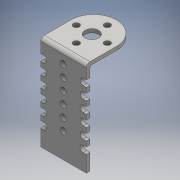
# Autodesk Inventor part: small motor mount
Saved by Autodesk Inventor 2016 (Build 200138000, 138)
## iProperties
Created: 2015-09-29
Part Number: small motor mount
Material: Generic
Document SubType Name: Modeling
Designer: Hulbert Office
Density: 1 g/cm^3
Appearance: Default
Author: Hulbert Office
Autodesk Inventor part; units mm, degrees
ref_plane "YZ Plane" through (0, 0, 0) normal (1, 0, 0) x (0, 1, 0)
ref_plane "XZ Plane" through (0, 0, 0) normal (0, 1, 0) x (-1, 0, 0)
ref_plane "XY Plane" through (0, 0, 0) normal (0, 0, 1) x (1, 0, 0)
sketch "Sketch1" plane through (0, 0, 0) normal (0, 1, 0) x (-1, 0, 0)
  line L0 (0, -52) -> (25, -52)
  line L1 (25, 0) -> (0, 0)
  line L2 (12.5, 0) -> (23.35, 0)
  line L3 (12.5, 0) -> (1.65, 0)
  line L4 (25, -11.25) -> (25, -14.1)
  line L5 (25, -23.95) -> (25, -26.8)
  line L6 (23.35, -7.75) -> (25, -7.75)
  line L7 (23.35, -11.25) -> (25, -11.25)
  arc A0 (23.35, -7.75) -> (23.35, -11.25) centre (23.35, -9.5) ccw
  line L8 (25, 0) -> (25, -7.75)
  arc A1 (23.35, -14.1) -> (23.35, -17.6) centre (23.35, -15.85) ccw
  arc A2 (23.35, -20.45) -> (23.35, -23.95) centre (23.35, -22.2) ccw
  arc A3 (23.35, -26.8) -> (23.35, -30.3) centre (23.35, -28.55) ccw
  arc A4 (23.35, -39.5) -> (23.35, -43) centre (23.35, -41.25) ccw
  line L9 (23.35, -39.5) -> (25, -39.5)
  line L10 (23.35, -43) -> (25, -43)
  line L11 (23.35, -36.65) -> (25, -36.65)
  line L12 (23.35, -33.15) -> (25, -33.15)
  line L13 (23.35, -23.95) -> (25, -23.95)
  line L14 (23.35, -20.45) -> (25, -20.45)
  line L15 (23.35, -17.6) -> (25, -17.6)
  line L16 (23.35, -14.1) -> (25, -14.1)
  line L17 (25, -17.6) -> (25, -20.45)
  line L18 (23.35, -26.8) -> (25, -26.8)
  line L19 (23.35, -30.3) -> (25, -30.3)
  line L20 (25, -43) -> (25, -52)
  line L21 (25, -36.65) -> (25, -39.5)
  arc A5 (23.35, -33.15) -> (23.35, -36.65) centre (23.35, -34.9) ccw
  line L22 (25, -30.3) -> (25, -33.15)
  line L23 (0, -11.25) -> (0, -14.1)
  line L24 (0, -23.95) -> (0, -26.8)
  line L25 (1.65, -7.75) -> (0, -7.75)
  line L26 (1.65, -11.25) -> (0, -11.25)
  arc A6 (1.65, -11.25) -> (1.65, -7.75) centre (1.65, -9.5) ccw
  line L27 (0, 0) -> (0, -7.75)
  arc A7 (1.65, -17.6) -> (1.65, -14.1) centre (1.65, -15.85) ccw
  arc A8 (1.65, -23.95) -> (1.65, -20.45) centre (1.65, -22.2) ccw
  arc A9 (1.65, -30.3) -> (1.65, -26.8) centre (1.65, -28.55) ccw
  arc A10 (1.65, -43) -> (1.65, -39.5) centre (1.65, -41.25) ccw
  line L28 (1.65, -39.5) -> (0, -39.5)
  line L29 (1.65, -43) -> (0, -43)
  line L30 (1.65, -36.65) -> (0, -36.65)
  line L31 (1.65, -33.15) -> (0, -33.15)
  line L32 (1.65, -23.95) -> (0, -23.95)
  line L33 (1.65, -20.45) -> (0, -20.45)
  line L34 (1.65, -17.6) -> (0, -17.6)
  line L35 (1.65, -14.1) -> (0, -14.1)
  line L36 (0, -17.6) -> (0, -20.45)
  line L37 (1.65, -26.8) -> (0, -26.8)
  line L38 (1.65, -30.3) -> (0, -30.3)
  line L39 (0, -43) -> (0, -52)
  line L40 (0, -36.65) -> (0, -39.5)
  arc A11 (1.65, -36.65) -> (1.65, -33.15) centre (1.65, -34.9) ccw
  line L41 (0, -30.3) -> (0, -33.15)
  circle A12 centre (12.5, -6.4) radius 1.65
  circle A13 centre (12.5, -12.75) radius 1.65
  circle A14 centre (12.5, -19.1) radius 1.65
  circle A15 centre (12.5, -25.45) radius 1.65
  circle A16 centre (12.5, -31.8) radius 1.65
  circle A17 centre (12.5, -38.15) radius 1.65
  dimension "d0" = 52
  dimension "d1" = 25
  dimension "d3" = 10.85
  dimension "d27" = 3.5
  dimension "d28" = 3.5
  dimension "d29" = 3.5
  dimension "d31" = 3.5
  dimension "d38" = 3.3
  dimension "d39" = 3.3
  dimension "d40" = 3.3
  dimension "d41" = 3.3
  dimension "d42" = 3.3
  dimension "d43" = 3.3
  constraints: 84 end point, 24 point on circle, 18 centre point, 12 tangent, 7 perpendicular, 2 point on line, 2 vertical, 1 midpoint
  measures "d0" distance of L1.end L0.start
  measures "d1" distance of L0.start L0.end
  measures "d3" distance of L2.start L2.end
  measures "d27" diameter of A1
  measures "d28" diameter of A2
  measures "d29" diameter of A3
  measures "d31" diameter of A4
  measures "d38" diameter of A12
  measures "d39" diameter of A13
  measures "d40" diameter of A14
  measures "d41" diameter of A15
  measures "d42" diameter of A16
  measures "d43" diameter of A17
extrude "Extrusion1" add sketch "Sketch1" along normal blind 2
sketch "Sketch2" plane through (0, 2, 0) normal (0, 1, 0) x (1, 0, 0)
  line L0 (-25, 7.75) -> (-25, 0) projected
  line L1 (-25, 0) -> (-25, 2)
  line L2 (-25, 2) -> (0, 2)
  line L3 (0, 0) -> (0, 7.75) projected
  line L4 (0, 2) -> (0, 0)
  line L5 (-25, 0) -> (0, 0) projected
  line L6 (0, 0) -> (-25, 0)
  dimension "d46" = 2
  constraints: 8 end point, 2 perpendicular, 1 collinear, 1 point on line
  measures "d46" distance of L0.end L1.end
extrude "Extrusion2" add sketch "Sketch2" along normal blind 27
fillet "Fillet1" radius 2 1 edges at (-12.5, 0, 0)
fillet "Fillet2" radius 1 1 edges at (-12.5, 2, -2)
sketch "Sketch3" plane through (-25, 29, 0) normal (0, 0, 1) x (1, 0, 0)
  line L0 (10.85, -27) -> (14.15, -27) projected
  line L1 (12.5, -27) -> (12.5, -13.5)
  circle A0 centre (12.5, -13.5) radius 3.75
  line L2 (12.5, -13.5) -> (21, -13.5)
  circle A1 centre (21, -13.5) radius 1.65
  circle A2 centre (12.5, -5) radius 1.65
  circle A3 centre (4, -13.5) radius 1.65
  circle A4 centre (12.5, -22) radius 1.65
  line L3 (25, -27) -> (25, 0) projected
  line L4 (0, -27) -> (0, 0) projected
  arc A5 (25, -13.5) -> (0, -13.5) centre (12.5, -12.537) ccw
  line L5 (0, -13.5) -> (-1.684, -13.0314)
  line L6 (-1.684, -13.0314) -> (-1.9019, 0.6389)
  line L7 (-1.9019, 0.6389) -> (9.9575, 0.6389)
  line L8 (9.9575, 0.6389) -> (27.127, 0.7206)
  line L9 (27.127, 0.7206) -> (26.6368, -13.7122)
  line L10 (26.6368, -13.7122) -> (25, -13.5)
  point P0 (25, -29)
  dimension "d51" = 13.5
  dimension "d52" = 7.5
  dimension "d53" = 8.5
  dimension "d54" = 3.3
  dimension "d57" = 360
  constraints: 16 end point, 6 centre point, 3 midpoint, 2 coincident, 2 point on circle, 1 horizontal, 1 perpendicular, 1 vertical, 9 other
  measures "d51" distance of L1.start L1.end
  measures "d52" diameter of A0
  measures "d53" distance of L2.start L2.end
  measures "d54" diameter of A1
extrude "Extrusion3" cut sketch "Sketch3" against normal blind 27 contours A5 L5 L6 L7 L8 L9 L10
extrude "Extrusion4" cut sketch "Sketch3" against normal blind 27 contours A4 L1 | L1 A4 | A1 | A2 | A3
extrude "Extrusion5" cut sketch "Sketch3" against normal blind 27 contours A0 L2 L1 | L1 L2 A0
body "Solid1"
